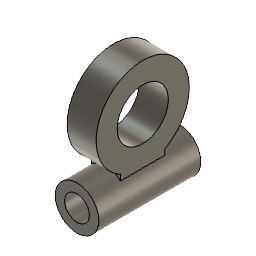
tube holder (Autodesk Fusion 360 design; units mm, degrees)
part number: 2026-01-13-14-52-33-679
Autodesk Fusion 360 part; units mm, degrees
sketch "Sketch1" plane through (0, 0, 0) normal (0, 1, 0) x (1, 0, 0)
  circle A0 centre (0, -3) radius 3
  circle A1 centre (0, -3) radius 1.7
  dimension "d1" = 3.4
  constraint concentric A0 A1
  measures "d1" diameter of A1
extrude "Extrude1" add sketch "Sketch1" along normal blind 14
sketch "Sketch2" plane through (0, 0, 0) normal (0, 0, 1) x (1, 0, 0)
ref_plane "WorkPlane1" through (0, 0, 6) normal (0, 0, 1) x (1, 0, 0)
sketch "Sketch3" plane through (0, 0, 6) normal (0, 0, 1) x (1, 0, 0)
  line L0 (-2, 10.0294) -> (2, 10.0294)
  line L1 (2, 10.0294) -> (2, 3.9745)
  line L2 (2, 3.9745) -> (-2, 3.9745)
  line L3 (-2, 3.9745) -> (-2, 10.0294)
  constraint horizontal L0
  constraint vertical L1
  constraint horizontal L2
  constraint vertical L3
extrude "Extrude2" add sketch "Sketch3" against normal blind 1
ref_plane "WorkPlane2" through (-2, 0, 0) normal (1, 0, 0) x (0, 1, 0)
sketch "Sketch4" plane through (-2, 0, 0) normal (1, 0, 0) x (0, 1, 0)
  circle A0 centre (7.0273, 11.6383) radius 6.3914
  circle A1 centre (7.0273, 11.6383) radius 3.5
  dimension "d8" = 7
  constraint concentric A0 A1
  measures "d8" diameter of A1
extrude "Extrude3" add sketch "Sketch4" along normal blind 4
